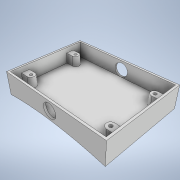
# Autodesk Inventor part: McCase
Saved by Autodesk Inventor 2021 (Build 250183000, 183)
## iProperties
Created: 2022-04-07
Part Number: McCase
Material: Generic
Document SubType Name: Modeling
Designer: Frederik
Density: 1 g/cm^3
Appearance: Default
Author: Frederik
Autodesk Inventor part; units mm, degrees
ref_plane "YZ Plane" through (0, 0, 0) normal (1, 0, 0) x (0, 1, 0)
ref_plane "XZ Plane" through (0, 0, 0) normal (0, 1, 0) x (-1, 0, 0)
sketch "Sketch4" plane through (0, 0, 0) normal (0, 0, 1) x (1, 0, 0)
  line L0 (0, 0) -> (200, 0) construction
  line L1 (0, 0) -> (200, 0) construction
  line L2 (100, 0) -> (100, 8)
  arc A0 (200, 0) -> (0, 0) centre (100, -621) ccw
  line L3 (0, 0) -> (0, 4)
  line L4 (200, 0) -> (200, 4)
  line L5 (100, 8) -> (100, 12)
  arc A1 (200, 4) -> (0, 4) centre (100, -617) ccw
  dimension "d11" = 200
  dimension "d13" = 8
  dimension "d14" = 4
  dimension "d15" = 4
  constraints: 12 end point, 6 point on circle, 4 vertical, 2 centre point, 2 horizontal, 1 collinear, 1 midpoint
  measures "d11" distance of L0.start L0.end
  measures "d13" distance of L2.start L2.end
  measures "d14" distance of L0.start L3.end
  measures "d15" distance of L2.end L5.end
extrude "Extrusion5" add sketch "Sketch4" against normal blind 150
sketch "Sketch5" plane through (0, 0, 0) normal (0, 0, 1) x (1, 0, 0)
  arc A0 (200, 4) -> (0, 4) centre (100, -617) ccw projected
  line L0 (100, 12) -> (100, 8)
  arc A1 (200, 0) -> (0, 0) centre (100, -621) ccw projected
  line L1 (0, 4) -> (200, 4)
  line L2 (200, 4) -> (200, 12)
  line L3 (200, 12) -> (0, 12)
  line L4 (0, 12) -> (0, 4)
  point P0 (200, 4)
  constraints: 10 end point, 2 parallel, 2 point on circle, 1 horizontal, 1 perpendicular, 1 vertical
extrude "Extrusion6" add sketch "Sketch5" against normal up to surface (150 mm away) contours A0 L3 L2 | A0 L4 L3
sketch "Sketch6" plane through (0, 12, 0) normal (0, 1, 0) x (1, 0, 0)
  line L0 (0, 0) -> (0, 150) projected
  line L1 (200, 0) -> (200, 150) projected
  line L2 (0, 150) -> (200, 150)
  line L3 (200, 150) -> (200, 0)
  line L4 (200, 0) -> (0, 0)
  line L5 (0, 0) -> (0, 150)
  line L6 (196, 4) -> (4, 4)
  line L7 (4, 4) -> (4, 146)
  line L8 (4, 146) -> (196, 146)
  line L9 (196, 146) -> (196, 4)
  dimension "d22" = 192
  dimension "d23" = 142
  constraints: 16 end point, 4 parallel, 2 horizontal, 2 perpendicular
  measures "d22" distance of L7.end L8.end
  measures "d23" distance of L6.end L7.end
extrude "Extrusion7" add sketch "Sketch6" along normal blind 30
sketch "Sketch7" plane through (0, 0, 0) normal (0, 0, 1) x (1, 0, 0)
  line L0 (196, 12) -> (4, 12) projected
  line L1 (100, 12) -> (100, 25) construction
  circle A0 centre (100, 25) radius 13
  point P0 (0, 0)
  dimension "d26" = 13
  dimension "d27" = 26
  constraints: 2 end point, 1 centre point, 1 coincident, 1 midpoint, 1 vertical
  measures "d26" distance of L1.start L1.end
  measures "d27" diameter of A0
extrude "Extrusion8" cut sketch "Sketch7" against normal up to surface (150 mm away)
sketch "Sketch8" plane through (4, 12, -4) normal (0, 1, 0) x (1, 0, 0)
  line L0 (192, 0) -> (192, 142) projected
  line L1 (192, 0) -> (192, 25)
  line L2 (96, 142) -> (0, 142) projected
  line L3 (0, 142) -> (0, 0) projected
  line L4 (192, 25) -> (177, 25)
  circle A0 centre (177, 25) radius 7.5
  line L5 (177, 32.5) -> (192, 32.5)
  line L6 (192, 32.5) -> (192, 17.5)
  line L7 (192, 17.5) -> (177, 17.5)
  line L8 (177, 17.5) -> (177, 32.5)
  line L9 (192, 0) -> (96, 0) construction
  line L10 (96, 0) -> (96, 71) construction
  line L11 (96, 71) -> (192, 71) construction
  line L12 (192, 71) -> (192, 0) construction
  point P0 (-4, -4)
  point P1 (177, 17.5)
  dimension "d33" = 15
  dimension "d30" = 25
  dimension "d32" = 15
  constraints: 20 end point, 4 parallel, 3 horizontal, 2 perpendicular, 2 point on line, 1 coincident, 3 other
  measures "d30" distance of L0.start L1.end
  measures "d32" distance of L1.end L4.end
extrude "Extrusion9" add sketch "Sketch8" along normal blind 20
sketch "Sketch9" plane through (4, 32, -4) normal (0, 1, 0) x (1, 0, 0)
  line L0 (192, 17.5) -> (177, 17.5) projected
  arc A0 (177, 32.5) -> (177, 17.5) centre (177, 25) ccw projected
  line L1 (177, 17.5) -> (177, 32.5)
  point P0 (-4, -4)
  constraints: 2 end point, 1 vertical
hole "Hole1" at (181, 32, -29) direction (0, -1, 0) diameter 6 end through all
pattern_circular "Circular Pattern1" count 2 over 360 about axis through (100, 2.6712, -75) along (0, 1, 0) of "Hole1", "Extrusion9"
ref_plane "Work Plane1" through (196, 42, -75) normal (0, 0, -1) x (-1, 0, 0)
mirror "Mirror1" about plane through (196, 42, -75) normal (0, 0, -1) of "Hole1", "Extrusion9", "Circular Pattern1"
body "Solid3"
